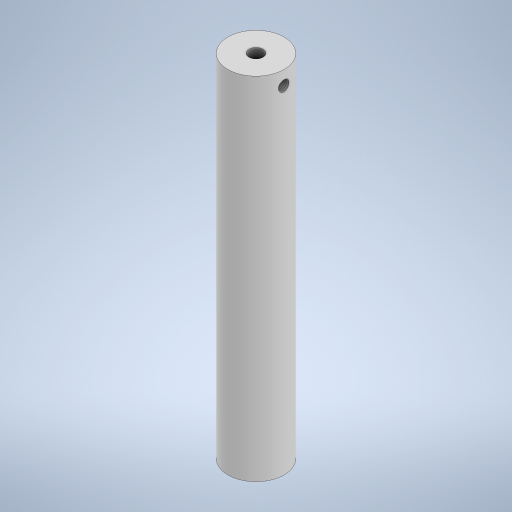
# Autodesk Inventor part: Вал
Saved by Autodesk Inventor 2023 (Build 270158000, 158)
## iProperties
Created: 2022-05-01
Part Number: Вал
Material: Типовые
Document SubType Name: Modeling
Designer: User
Density: 1 g/cm^3
Appearance: По умолчанию
Author: User
Autodesk Inventor part; units mm, degrees
ref_plane "YZ Plane" through (0, 0, 0) normal (1, 0, 0) x (0, 1, 0)
ref_plane "XZ Plane" through (0, 0, 0) normal (0, 1, 0) x (-1, 0, 0)
ref_plane "XY Plane" through (0, 0, 0) normal (0, 0, 1) x (1, 0, 0)
sketch "Эскиз1" plane through (0, 0, 0) normal (0, 1, 0) x (-1, 0, 0)
  circle A0 centre (0, 0) radius 8
  dimension "d0" = 16
  constraints: 1 centre point, 1 coincident
  measures "d0" diameter of A0
extrude "Выдавливание1" add sketch "Эскиз1" along normal blind 100
sketch "Эскиз2" plane through (0, 0, 0) normal (0, -1, 0) x (1, 0, 0)
  circle A0 centre (0, 0) radius 22.5
  line L0 (0, 0) -> (0, 4.5)
  line L1 (0, 0) -> (0, -4.5)
  dimension "d3" = 45
  dimension "d4" = 4.5
  dimension "d5" = 4.5
  constraints: 4 end point, 2 vertical, 1 centre point, 1 coincident
  measures "d3" diameter of A0
  measures "d4" distance of L0.start L0.end
  measures "d5" distance of L0.start L1.end
hole "Отверстие1" at (0, 0, 4.5) at (0, 0, -4.5) direction (0, 1, 0) diameter 2.459 depth 8 tip angle 118 thread size "M3x0.5" class "6H" standard "ISO Metric profile"
chamfer "Фаска1" distance 0.5 angle 45 2 edges at (0, 0, 5.7295) (0, 0, -3.2705)
sketch "Эскиз3" plane through (0, 100, 0) normal (0, 1, 0) x (1, 0, 0)
  circle A0 centre (0, 0) radius 2
  dimension "d16" = 4
  constraints: 1 centre point, 1 coincident
  measures "d16" diameter of A0
extrude "Выдавливание2" cut sketch "Эскиз3" against normal blind 10
sketch "Эскиз4" plane through (0, 0, 0) normal (1, 0, 0) x (0, 1, 0)
  line L0 (100, -8) -> (100, 8) projected
  line L1 (100, 0) -> (96, 0)
  circle A0 centre (96, 0) radius 1.5
  point P0 (0, 0)
  dimension "d29" = 4
  dimension "d30" = 3
  constraints: 2 end point, 1 centre point, 1 coincident, 1 horizontal, 1 midpoint
  measures "d29" distance of L1.start L1.end
  measures "d30" diameter of A0
extrude "Выдавливание3" cut sketch "Эскиз4" along normal mid plane 30.75
thread "Резьба1" size "M3x0.5" class "6H" standard "ISO Metric profile" full length
